Autodesk Fusion 360 part; units mm, degrees
(part 4 of 18)
  spline S17 degree 5 poles (4.4666, -33.3018) (4.4679, -33.2978) (4.4703, -33.2898) (4.474, -33.2778) (4.4789, -33.2619) (4.485, -33.242) (4.491, -33.2221) (4.497, -33.2023) (4.503, -33.1825) (4.5089, -33.1627) (4.5147, -33.1429) (4.5206, -33.1232) (4.5263, -33.1036) (4.5321, -33.0839) (4.5378, -33.0643) (4.5434, -33.0447) (4.549, -33.0252) (4.5546, -33.0057) (4.5601, -32.9862) (4.5656, -32.9667) (4.5711, -32.9473) (4.5765, -32.928) (4.5818, -32.9086) (4.5872, -32.8893) (4.5924, -32.87) (4.5977, -32.8508) (4.6029, -32.8316) (4.608, -32.8125) (4.6132, -32.7933) (4.6182, -32.7742) (4.6233, -32.7552) (4.6283, -32.7362) (4.6332, -32.7172) (4.6381, -32.6982) (4.643, -32.6793) (4.6478, -32.6605) (4.6526, -32.6416) (4.6574, -32.6228) (4.6621, -32.6041) (4.6667, -32.5854) (4.6714, -32.5667) (4.676, -32.5481) (4.6805, -32.5295) (4.685, -32.5109) (4.6895, -32.4924) (4.6939, -32.4739) (4.6983, -32.4555) (4.7026, -32.4371) (4.707, -32.4187) (4.7112, -32.4004) (4.7154, -32.3821) (4.7196, -32.3639) (4.7238, -32.3457) (4.7279, -32.3275) (4.732, -32.3094) (4.736, -32.2913) (4.74, -32.2733) (4.7439, -32.2553) (4.7478, -32.2374) (4.7517, -32.2195) (4.7555, -32.2016) (4.7593, -32.1838) (4.7631, -32.166) (4.7668, -32.1483) (4.7705, -32.1306) (4.7741, -32.113) (4.7777, -32.0954) (4.7813, -32.0779) (4.7848, -32.0604) (4.7883, -32.0429) (4.7917, -32.0255) (4.7951, -32.0081) (4.7985, -31.9908) (4.8018, -31.9736) (4.8051, -31.9563) (4.8083, -31.9392) (4.8115, -31.922) (4.8147, -31.905) (4.8179, -31.8879) (4.821, -31.871) (4.824, -31.854) (4.827, -31.8371) (4.83, -31.8203) (4.833, -31.8035) (4.8359, -31.7868) (4.8387, -31.7701) (4.8416, -31.7535) (4.8444, -31.7369) (4.8471, -31.7204) (4.8499, -31.7039) (4.8526, -31.6874) (4.8552, -31.6711) (4.8578, -31.6548) (4.8604, -31.6385) (4.8629, -31.6223) (4.8654, -31.6061) (4.8679, -31.59) (4.8703, -31.5739) (4.8727, -31.5579) (4.8751, -31.542) (4.8774, -31.5261) (4.8797, -31.5103) (4.882, -31.4945) (4.8842, -31.4787) (4.8864, -31.4631) (4.8885, -31.4475) (4.8906, -31.4319) (4.8927, -31.4164) (4.8947, -31.401) (4.8967, -31.3856) (4.8987, -31.3703) (4.9006, -31.355) (4.9026, -31.3398) (4.9044, -31.3247) (4.9063, -31.3096) (4.908, -31.2946) (4.9098, -31.2796) (4.9115, -31.2647) (4.9132, -31.2499) (4.9149, -31.2351) (4.9165, -31.2204) (4.9181, -31.2057) (4.9197, -31.1911) (4.9212, -31.1766) (4.9227, -31.1621) (4.9242, -31.1477) (4.9256, -31.1334) (4.927, -31.1191) (4.9284, -31.1049) (4.9297, -31.0908) (4.931, -31.0767) (4.9323, -31.0627) (4.9335, -31.0488) (4.9347, -31.0349) (4.9359, -31.0211) (4.9371, -31.0074) (4.9382, -30.9938) (4.9393, -30.9802) (4.9403, -30.9667) (4.9413, -30.9532) (4.9423, -30.9398) (4.9433, -30.9265) (4.9442, -30.9133) (4.9451, -30.9002) (4.946, -30.8871) (4.9468, -30.8741) (4.9476, -30.8611) (4.9484, -30.8483) (4.9492, -30.8355) (4.9499, -30.8228) (4.9506, -30.8102) (4.9513, -30.7976) (4.9519, -30.7851) (4.9525, -30.7727) (4.9531, -30.7604) (4.9537, -30.7482) (4.9542, -30.736) (4.9547, -30.724) (4.9552, -30.712) (4.9556, -30.7001) (4.9561, -30.6882) (4.9565, -30.6765) (4.9568, -30.6648) (4.9572, -30.6533) (4.9575, -30.6418) (4.9578, -30.6304) (4.9581, -30.6191) (4.9583, -30.6078) (4.9585, -30.5967) (4.9587, -30.5856) (4.9589, -30.5747) (4.9591, -30.5638) (4.9592, -30.553) (4.9593, -30.5424) (4.9594, -30.5318) (4.9594, -30.5213) (4.9595, -30.5109) (4.9595, -30.5006) (4.9595, -30.4904) (4.9595, -30.4802) (4.9594, -30.4702) (4.9594, -30.4603) (4.9593, -30.4505) (4.9592, -30.4408) (4.9591, -30.4312) (4.9589, -30.4217) (4.9588, -30.4122) (4.9586, -30.4029) (4.9584, -30.3938) (4.9582, -30.3847) (4.9579, -30.3757) (4.9577, -30.3668) (4.9574, -30.3581) (4.9572, -30.3494) (4.9569, -30.3409) (4.9566, -30.3324) (4.9562, -30.3241) (4.9559, -30.3159) (4.9556, -30.3079) (4.9552, -30.2999) (4.9548, -30.2921) (4.9545, -30.2844) (4.9541, -30.2768) (4.9537, -30.2693) (4.9532, -30.262) (4.9528, -30.2547) (4.9524, -30.2477) (4.9519, -30.2407) (4.9515, -30.2339) (4.951, -30.2272) (4.9506, -30.2206) (4.9501, -30.2142) (4.9496, -30.2079) (4.9492, -30.2018) (4.9487, -30.1958) (4.9482, -30.1899) (4.9477, -30.1842) (4.9472, -30.1787) (4.9468, -30.1733) (4.9463, -30.168) (4.9458, -30.1629) (4.9453, -30.158) (4.9448, -30.1532) (4.9444, -30.1486) (4.9439, -30.1441) (4.9434, -30.1398) (4.943, -30.1357) (4.9426, -30.1317) (4.9421, -30.128) (4.9417, -30.1244) (4.9413, -30.121) (4.9409, -30.1177) (4.9405, -30.1147) (4.9401, -30.1119) (4.9398, -30.1092) (4.9395, -30.1068) (4.9392, -30.1045) (4.9389, -30.1025) (4.9386, -30.1006) (4.9384, -30.099) (4.9382, -30.0976) (4.9381, -30.0967) (4.938, -30.0961) (4.9379, -30.0958) (4.9379, -30.0956) knots -1 -1 -1 -1 -1 -1 -0.99583333 -0.99166667 -0.9875 -0.98333333 -0.97916667 -0.975 -0.97083333 -0.96666667 -0.9625 -0.95833333 -0.95416667 -0.95 -0.94583333 -0.94166667 -0.9375 -0.93333333 -0.92916667 -0.925 -0.92083333 -0.91666667 -0.9125 -0.90833333 -0.90416667 -0.9 -0.89583333 -0.89166667 -0.8875 -0.88333333 -0.87916667 -0.875 -0.87083333 -0.86666667 -0.8625 -0.85833333 -0.85416667 -0.85 -0.84583333 -0.84166667 -0.8375 -0.83333333 -0.82916667 -0.825 -0.82083333 -0.81666667 -0.8125 -0.80833333 -0.80416667 -0.8 -0.79583333 -0.79166667 -0.7875 -0.78333333 -0.77916667 -0.775 -0.77083333 -0.76666667 -0.7625 -0.75833333 -0.75416667 -0.75 -0.74583333 -0.74166667 -0.7375 -0.73333333 -0.72916667 -0.725 -0.72083333 -0.71666667 -0.7125 -0.70833333 -0.70416667 -0.7 -0.69583333 -0.69166667 -0.6875 -0.68333333 -0.67916667 -0.675 -0.67083333 -0.66666667 -0.6625 -0.65833333 -0.65416667 -0.65 -0.64583333 -0.64166667 -0.6375 -0.63333333 -0.62916667 -0.625 -0.62083333 -0.61666667 -0.6125 -0.60833333 -0.60416667 -0.6 -0.59583333 -0.59166667 -0.5875 -0.58333333 -0.57916667 -0.575 -0.57083333 -0.56666667 -0.5625 -0.55833333 -0.55416667 -0.55 -0.54583333 -0.54166667 -0.5375 -0.53333333 -0.52916667 -0.525 -0.52083333 -0.51666667 -0.5125 -0.50833333 -0.50416667 -0.5 -0.49583333 -0.49166667 -0.4875 -0.48333333 -0.47916667 -0.475 -0.47083333 -0.46666667 -0.4625 -0.45833333 -0.45416667 -0.45 -0.44583333 -0.44166667 -0.4375 -0.43333333 -0.42916667 -0.425 -0.42083333 -0.41666667 -0.4125 -0.40833333 -0.40416667 -0.4 -0.39583333 -0.39166667 -0.3875 -0.38333333 -0.37916667 -0.375 -0.37083333 -0.36666667 -0.3625 -0.35833333 -0.35416667 -0.35 -0.34583333 -0.34166667 -0.3375 -0.33333333 -0.32916667 -0.325 -0.32083333 -0.31666667 -0.3125 -0.30833333 -0.30416667 -0.3 -0.29583333 -0.29166667 -0.2875 -0.28333333 -0.27916667 -0.275 -0.27083333 -0.26666667 -0.2625 -0.25833333 -0.25416667 -0.25 -0.24583333 -0.24166667 -0.2375 -0.23333333 -0.22916667 -0.225 -0.22083333 -0.21666667 -0.2125 -0.20833333 -0.20416667 -0.2 -0.19583333 -0.19166667 -0.1875 -0.18333333 -0.17916667 -0.175 -0.17083333 -0.16666667 -0.1625 -0.15833333 -0.15416667 -0.15 -0.14583333 -0.14166667 -0.1375 -0.13333333 -0.12916667 -0.125 -0.12083333 -0.11666667 -0.1125 -0.10833333 -0.10416667 -0.1 -0.09583333 -0.09166667 -0.0875 -0.08333333 -0.07916667 -0.075 -0.07083333 -0.06666667 -0.0625 -0.05833333 -0.05416667 -0.05 -0.04583333 -0.04166667 -0.0375 -0.03333333 -0.02916667 -0.025 -0.02083333 -0.01666667 -0.0125 -0.00833333 -0.00416667 0 0 0 0 0 0
  line L34 (4.9379, -30.0956) -> (4.9377, -30.0943)
  line L35 (4.9377, -30.0943) -> (4.6751, -28.494)
  arc A18 (4.6751, -28.494) -> (7.3186, -27.9321) centre (0, 0) ccw
  line L36 (7.3186, -27.9321) -> (7.7297, -29.5008)
  line L37 (7.7297, -29.5008) -> (7.73, -29.5021)
  spline S18 degree 5 poles (7.73, -29.5021) (7.7301, -29.5023) (7.7301, -29.5026) (7.7303, -29.5032) (7.7306, -29.5041) (7.7309, -29.5055) (7.7314, -29.507) (7.7319, -29.5088) (7.7325, -29.5108) (7.7331, -29.513) (7.7338, -29.5153) (7.7345, -29.5179) (7.7354, -29.5206) (7.7363, -29.5236) (7.7372, -29.5267) (7.7382, -29.53) (7.7393, -29.5334) (7.7404, -29.537) (7.7416, -29.5408) (7.7429, -29.5448) (7.7442, -29.5489) (7.7456, -29.5531) (7.7471, -29.5576) (7.7486, -29.5621) (7.7502, -29.5668) (7.7518, -29.5717) (7.7535, -29.5767) (7.7552, -29.5818) (7.7571, -29.5871) (7.7589, -29.5925) (7.7609, -29.598) (7.7629, -29.6037) (7.765, -29.6095) (7.7671, -29.6155) (7.7693, -29.6215) (7.7715, -29.6277) (7.7738, -29.634) (7.7762, -29.6404) (7.7786, -29.6469) (7.7811, -29.6536) (7.7836, -29.6603) (7.7862, -29.6672) (7.7889, -29.6742) (7.7916, -29.6813) (7.7944, -29.6885) (7.7973, -29.6958) (7.8002, -29.7032) (7.8032, -29.7107) (7.8062, -29.7184) (7.8093, -29.7261) (7.8124, -29.7339) (7.8156, -29.7418) (7.8189, -29.7498) (7.8222, -29.7579) (7.8256, -29.7661) (7.829, -29.7744) (7.8325, -29.7828) (7.8361, -29.7913) (7.8397, -29.7999) (7.8434, -29.8085) (7.8471, -29.8173) (7.8509, -29.8261) (7.8548, -29.835) (7.8587, -29.844) (7.8627, -29.8531) (7.8667, -29.8623) (7.8708, -29.8715) (7.875, -29.8809) (7.8792, -29.8903) (7.8834, -29.8998) (7.8878, -29.9093) (7.8922, -29.919) (7.8966, -29.9287) (7.9011, -29.9385) (7.9057, -29.9483) (7.9103, -29.9583) (7.9149, -29.9683) (7.9197, -29.9784) (7.9245, -29.9885) (7.9293, -29.9988) (7.9342, -30.0091) (7.9392, -30.0194) (7.9442, -30.0298) (7.9493, -30.0403) (7.9544, -30.0509) (7.9596, -30.0615) (7.9649, -30.0722) (7.9702, -30.083) (7.9756, -30.0938) (7.981, -30.1047) (7.9865, -30.1157) (7.992, -30.1267) (7.9976, -30.1378) (8.0033, -30.1489) (8.009, -30.1601) (8.0148, -30.1713) (8.0206, -30.1826) (8.0265, -30.194) (8.0325, -30.2054) (8.0385, -30.2169) (8.0445, -30.2285) (8.0506, -30.2401) (8.0568, -30.2517) (8.063, -30.2634) (8.0693, -30.2752) (8.0757, -30.287) (8.0821, -30.2989) (8.0885, -30.3108) (8.0951, -30.3228) (8.1016, -30.3348) (8.1083, -30.3468) (8.1149, -30.359) (8.1217, -30.3711) (8.1285, -30.3834) (8.1353, -30.3956) (8.1422, -30.408) (8.1492, -30.4203) (8.1562, -30.4327) (8.1633, -30.4452) (8.1705, -30.4577) (8.1776, -30.4703) (8.1849, -30.4829) (8.1922, -30.4955) (8.1996, -30.5082) (8.207, -30.521) (8.2145, -30.5337) (8.222, -30.5466) (8.2296, -30.5594) (8.2372, -30.5723) (8.2449, -30.5853) (8.2527, -30.5983) (8.2605, -30.6113) (8.2683, -30.6244) (8.2763, -30.6375) (8.2842, -30.6507) (8.2923, -30.6639) (8.3004, -30.6771) (8.3085, -30.6904) (8.3167, -30.7037) (8.325, -30.717) (8.3333, -30.7304) (8.3416, -30.7438) (8.3501, -30.7573) (8.3585, -30.7708) (8.3671, -30.7843) (8.3757, -30.7979) (8.3843, -30.8115) (8.393, -30.8252) (8.4017, -30.8388) (8.4106, -30.8526) (8.4194, -30.8663) (8.4283, -30.8801) (8.4373, -30.8939) (8.4463, -30.9078) (8.4554, -30.9216) (8.4646, -30.9356) (8.4737, -30.9495) (8.483, -30.9635) (8.4923, -30.9775) (8.5016, -30.9915) (8.5111, -31.0056) (8.5205, -31.0197) (8.53, -31.0338) (8.5396, -31.048) (8.5492, -31.0622) (8.5589, -31.0764) (8.5687, -31.0907) (8.5785, -31.105) (8.5883, -31.1193) (8.5982, -31.1336) (8.6082, -31.148) (8.6182, -31.1624) (8.6282, -31.1768) (8.6383, -31.1912) (8.6485, -31.2057) (8.6587, -31.2202) (8.669, -31.2348) (8.6794, -31.2493) (8.6897, -31.2639) (8.7002, -31.2785) (8.7107, -31.2931) (8.7212, -31.3078) (8.7318, -31.3225) (8.7425, -31.3372) (8.7532, -31.3519) (8.7639, -31.3667) (8.7748, -31.3814) (8.7856, -31.3962) (8.7966, -31.4111) (8.8075, -31.4259) (8.8186, -31.4408) (8.8296, -31.4557) (8.8408, -31.4706) (8.852, -31.4855) (8.8632, -31.5005) (8.8745, -31.5154) (8.8859, -31.5304) (8.8973, -31.5455) (8.9087, -31.5605) (8.9202, -31.5756) (8.9318, -31.5907) (8.9434, -31.6058) (8.9551, -31.6209) (8.9668, -31.636) (8.9786, -31.6512) (8.9904, -31.6664) (9.0023, -31.6816) (9.0142, -31.6968) (9.0262, -31.712) (9.0382, -31.7273) (9.0503, -31.7425) (9.0624, -31.7578) (9.0746, -31.7731) (9.0869, -31.7885) (9.0992, -31.8038) (9.1115, -31.8192) (9.1239, -31.8345) (9.1364, -31.8499) (9.1489, -31.8653) (9.1614, -31.8808) (9.174, -31.8962) (9.1867, -31.9117) (9.1994, -31.9271) (9.2122, -31.9426) (9.225, -31.9581) (9.2379, -31.9736) (9.2508, -31.9892) (9.2638, -32.0047) (9.2768, -32.0203) (9.2899, -32.0358) (9.303, -32.0514) (9.3162, -32.067) (9.3294, -32.0826) (9.3427, -32.0982) (9.356, -32.1139) (9.3694, -32.1295) (9.3829, -32.1452) (9.3964, -32.1609) (9.4099, -32.1766) (9.4235, -32.1923) (9.4371, -32.208) (9.4481, -32.2206) (9.4563, -32.23) (9.4618, -32.2363) (9.4646, -32.2394) knots 0 0 0 0 0 0 0.00416667 0.00833333 0.0125 0.01666667 0.02083333 0.025 0.02916667 0.03333333 0.0375 0.04166667 0.04583333 0.05 0.05416667 0.05833333 0.0625 0.06666667 0.07083333 0.075 0.07916667 0.08333333 0.0875 0.09166667 0.09583333 0.1 0.10416667 0.10833333 0.1125 0.11666667 0.12083333 0.125 0.12916667 0.13333333 0.1375 0.14166667 0.14583333 0.15 0.15416667 0.15833333 0.1625 0.16666667 0.17083333 0.175 0.17916667 0.18333333 0.1875 0.19166667 0.19583333 0.2 0.20416667 0.20833333 0.2125 0.21666667 0.22083333 0.225 0.22916667 0.23333333 0.2375 0.24166667 0.24583333 0.25 0.25416667 0.25833333 0.2625 0.26666667 0.27083333 0.275 0.27916667 0.28333333 0.2875 0.29166667 0.29583333 0.3 0.30416667 0.30833333 0.3125 0.31666667 0.32083333 0.325 0.32916667 0.33333333 0.3375 0.34166667 0.34583333 0.35 0.35416667 0.35833333 0.3625 0.36666667 0.37083333 0.375 0.37916667 0.38333333 0.3875 0.39166667 0.39583333 0.4 0.40416667 0.40833333 0.4125 0.41666667 0.42083333 0.425 0.42916667 0.43333333 0.4375 0.44166667 0.44583333 0.45 0.45416667 0.45833333 0.4625 0.46666667 0.47083333 0.475 0.47916667 0.48333333 0.4875 0.49166667 0.49583333 0.5 0.50416667 0.50833333 0.5125 0.51666667 0.52083333 0.525 0.52916667 0.53333333 0.5375 0.54166667 0.54583333 0.55 0.55416667 0.55833333 0.5625 0.56666667 0.57083333 0.575 0.57916667 0.58333333 0.5875 0.59166667 0.59583333 0.6 0.60416667 0.60833333 0.6125 0.61666667 0.62083333 0.625 0.62916667 0.63333333 0.6375 0.64166667 0.64583333 0.65 0.65416667 0.65833333 0.6625 0.66666667 0.67083333 0.675 0.67916667 0.68333333 0.6875 0.69166667 0.69583333 0.7 0.70416667 0.70833333 0.7125 0.71666667 0.72083333 0.725 0.72916667 0.73333333 0.7375 0.74166667 0.74583333 0.75 0.75416667 0.75833333 0.7625 0.76666667 0.77083333 0.775 0.77916667 0.78333333 0.7875 0.79166667 0.79583333 0.8 0.80416667 0.80833333 0.8125 0.81666667 0.82083333 0.825 0.82916667 0.83333333 0.8375 0.84166667 0.84583333 0.85 0.85416667 0.85833333 0.8625 0.86666667 0.87083333 0.875 0.87916667 0.88333333 0.8875 0.89166667 0.89583333 0.9 0.90416667 0.90833333 0.9125 0.91666667 0.92083333 0.925 0.92916667 0.93333333 0.9375 0.94166667 0.94583333 0.95 0.95416667 0.95833333 0.9625 0.96666667 0.97083333 0.975 0.97916667 0.98333333 0.9875 0.99166667 0.99583333 1 1 1 1 1 1
  arc A19 (9.4646, -32.2394) -> (11.2929, -31.6454) centre (0, 0) ccw
  spline S19 degree 5 poles (11.2929, -31.6454) (11.2932, -31.6412) (11.294, -31.6329) (11.2951, -31.6204) (11.2966, -31.6038) (11.2984, -31.5831) (11.3001, -31.5624) (11.3019, -31.5417) (11.3036, -31.5211) (11.3052, -31.5006) (11.3069, -31.48) (11.3085, -31.4595) (11.31, -31.4391) (11.3116, -31.4187) (11.3131, -31.3983) (11.3145, -31.378) (11.3159, -31.3577) (11.3173, -31.3375) (11.3187, -31.3173) (11.32, -31.2971) (11.3213, -31.277) (11.3226, -31.2569) (11.3238, -31.2369) (11.325, -31.2169) (11.3262, -31.1969) (11.3273, -31.177) (11.3284, -31.1572) (11.3294, -31.1374) (11.3305, -31.1176) (11.3315, -31.0979) (11.3324, -31.0782) (11.3334, -31.0585) (11.3343, -31.0389) (11.3351, -31.0194) (11.336, -30.9999) (11.3368, -30.9804) (11.3375, -30.961) (11.3383, -30.9416) (11.339, -30.9223) (11.3397, -30.903) (11.3403, -30.8838) (11.3409, -30.8646) (11.3415, -30.8455) (11.342, -30.8264) (11.3426, -30.8073) (11.343, -30.7884) (11.3435, -30.7694) (11.3439, -30.7505) (11.3443, -30.7316) (11.3447, -30.7128) (11.345, -30.6941) (11.3453, -30.6754) (11.3456, -30.6567) (11.3458, -30.6381) (11.3461, -30.6195) (11.3462, -30.601) (11.3464, -30.5826) (11.3465, -30.5642) (11.3466, -30.5458) (11.3467, -30.5275) (11.3467, -30.5092) (11.3467, -30.491) (11.3467, -30.4728) (11.3466, -30.4547) (11.3466, -30.4367) (11.3464, -30.4187) (11.3463, -30.4007) (11.3461, -30.3828) (11.3459, -30.365) (11.3457, -30.3472) (11.3455, -30.3294) (11.3452, -30.3117) (11.3449, -30.2941) (11.3445, -30.2765) (11.3442, -30.259) (11.3438, -30.2415) (11.3434, -30.2241) (11.3429, -30.2067) (11.3424, -30.1894) (11.3419, -30.1722) (11.3414, -30.155) (11.3409, -30.1378) (11.3403, -30.1207) (11.3397, -30.1037) (11.339, -30.0867) (11.3384, -30.0698) (11.3377, -30.053) (11.337, -30.0362) (11.3363, -30.0194) (11.3355, -30.0027) (11.3347, -29.9861) (11.3339, -29.9695) (11.3331, -29.953) (11.3322, -29.9366) (11.3313, -29.9202) (11.3304, -29.9038) (11.3295, -29.8876) (11.3285, -29.8714) (11.3275, -29.8552) (11.3265, -29.8391) (11.3255, -29.8231) (11.3244, -29.8071) (11.3234, -29.7912) (11.3222, -29.7754) (11.3211, -29.7596) (11.32, -29.7439) (11.3188, -29.7282) (11.3176, -29.7126) (11.3164, -29.6971) (11.3152, -29.6817) (11.3139, -29.6663) (11.3126, -29.6509) (11.3113, -29.6357) (11.31, -29.6205) (11.3087, -29.6053) (11.3073, -29.5903) (11.3059, -29.5753) (11.3045, -29.5603) (11.3031, -29.5454) (11.3016, -29.5306) (11.3002, -29.5159) (11.2987, -29.5013) (11.2972, -29.4867) (11.2957, -29.4721) (11.2941, -29.4577) (11.2926, -29.4433) (11.291, -29.429) (11.2894, -29.4147) (11.2878, -29.4006) (11.2861, -29.3865) (11.2845, -29.3724) (11.2828, -29.3585) (11.2811, -29.3446) (11.2794, -29.3308) (11.2777, -29.317) (11.276, -29.3034) (11.2742, -29.2898) (11.2725, -29.2763) (11.2707, -29.2628) (11.2689, -29.2495) (11.2671, -29.2362) (11.2653, -29.223) (11.2634, -29.2098) (11.2616, -29.1968) (11.2597, -29.1838) (11.2578, -29.1709) (11.2559, -29.1581) (11.254, -29.1453) (11.2521, -29.1327) (11.2502, -29.1201) (11.2482, -29.1076) (11.2463, -29.0952) (11.2443, -29.0829) (11.2423, -29.0706) (11.2403, -29.0584) (11.2383, -29.0464) (11.2363, -29.0344) (11.2343, -29.0224) (11.2323, -29.0106) (11.2302, -28.9989) (11.2282, -28.9872) (11.2261, -28.9756) (11.2241, -28.9642) (11.222, -28.9528) (11.2199, -28.9415) (11.2179, -28.9302) (11.2158, -28.9191) (11.2137, -28.9081) (11.2116, -28.8971) (11.2095, -28.8863) (11.2074, -28.8755) (11.2053, -28.8649) (11.2032, -28.8543) (11.201, -28.8438) (11.1989, -28.8335) (11.1968, -28.8232) (11.1947, -28.813) (11.1926, -28.8029) (11.1904, -28.7929) (11.1883, -28.783) (11.1862, -28.7733) (11.1841, -28.7636) (11.1819, -28.754) (11.1798, -28.7445) (11.1777, -28.7351) (11.1756, -28.7259) (11.1735, -28.7167) (11.1714, -28.7076) (11.1693, -28.6987) (11.1672, -28.6898) (11.1651, -28.6811) (11.163, -28.6725) (11.1609, -28.6639) (11.1588, -28.6555) (11.1568, -28.6473) (11.1547, -28.6391) (11.1527, -28.631) (11.1507, -28.6231) (11.1486, -28.6153) (11.1466, -28.6075) (11.1446, -28.6) (11.1427, -28.5925) (11.1407, -28.5851) (11.1387, -28.5779) (11.1368, -28.5708) (11.1349, -28.5639) (11.133, -28.557) (11.1311, -28.5503) (11.1293, -28.5437) (11.1274, -28.5373) (11.1256, -28.531) (11.1238, -28.5248) (11.1221, -28.5187) (11.1203, -28.5128) (11.1186, -28.5071) (11.1169, -28.5014) (11.1153, -28.496) (11.1136, -28.4906) (11.112, -28.4854) (11.1105, -28.4804) (11.1089, -28.4755) (11.1074, -28.4708) (11.106, -28.4662) (11.1046, -28.4618) (11.1032, -28.4575) (11.1018, -28.4534) (11.1005, -28.4495) (11.0993, -28.4457) (11.0981, -28.4421) (11.0969, -28.4387) (11.0958, -28.4354) (11.0948, -28.4323) (11.0937, -28.4294) (11.0928, -28.4267) (11.0919, -28.4242) (11.0911, -28.4219) (11.0903, -28.4197) (11.0896, -28.4178) (11.089, -28.4161) (11.0884, -28.4145) (11.0879, -28.4132) (11.0876, -28.4124) (11.0874, -28.4118) (11.0873, -28.4115) (11.0872, -28.4113) knots -1 -1 -1 -1 -1 -1 -0.99583333 -0.99166667 -0.9875 -0.98333333 -0.97916667 -0.975 -0.97083333 -0.96666667 -0.9625 -0.95833333 -0.95416667 -0.95 -0.94583333 -0.94166667 -0.9375 -0.93333333 -0.92916667 -0.925 -0.92083333 -0.91666667 -0.9125 -0.90833333 -0.90416667 -0.9 -0.89583333 -0.89166667 -0.8875 -0.88333333 -0.87916667 -0.875 -0.87083333 -0.86666667 -0.8625 -0.85833333 -0.85416667 -0.85 -0.84583333 -0.84166667 -0.8375 -0.83333333 -0.82916667 -0.825 -0.82083333 -0.81666667 -0.8125 -0.80833333 -0.80416667 -0.8 -0.79583333 -0.79166667 -0.7875 -0.78333333 -0.77916667 -0.775 -0.77083333 -0.76666667 -0.7625 -0.75833333 -0.75416667 -0.75 -0.74583333 -0.74166667 -0.7375 -0.73333333 -0.72916667 -0.725 -0.72083333 -0.71666667 -0.7125 -0.70833333 -0.70416667 -0.7 -0.69583333 -0.69166667 -0.6875 -0.68333333 -0.67916667 -0.675 -0.67083333 -0.66666667 -0.6625 -0.65833333 -0.65416667 -0.65 -0.64583333 -0.64166667 -0.6375 -0.63333333 -0.62916667 -0.625 -0.62083333 -0.61666667 -0.6125 -0.60833333 -0.60416667 -0.6 -0.59583333 -0.59166667 -0.5875 -0.58333333 -0.57916667 -0.575 -0.57083333 -0.56666667 -0.5625 -0.55833333 -0.55416667 -0.55 -0.54583333 -0.54166667 -0.5375 -0.53333333 -0.52916667 -0.525 -0.52083333 -0.51666667 -0.5125 -0.50833333 -0.50416667 -0.5 -0.49583333 -0.49166667 -0.4875 -0.48333333 -0.47916667 -0.475 -0.47083333 -0.46666667 -0.4625 -0.45833333 -0.45416667 -0.45 -0.44583333 -0.44166667 -0.4375 -0.43333333 -0.42916667 -0.425 -0.42083333 -0.41666667 -0.4125 -0.40833333 -0.40416667 -0.4 -0.39583333 -0.39166667 -0.3875 -0.38333333 -0.37916667 -0.375 -0.37083333 -0.36666667 -0.3625 -0.35833333 -0.35416667 -0.35 -0.34583333 -0.34166667 -0.3375 -0.33333333 -0.32916667 -0.325 -0.32083333 -0.31666667 -0.3125 -0.30833333 -0.30416667 -0.3 -0.29583333 -0.29166667 -0.2875 -0.28333333 -0.27916667 -0.275 -0.27083333 -0.26666667 -0.2625 -0.25833333 -0.25416667 -0.25 -0.24583333 -0.24166667 -0.2375 -0.23333333 -0.22916667 -0.225 -0.22083333 -0.21666667 -0.2125 -0.20833333 -0.20416667 -0.2 -0.19583333 -0.19166667 -0.1875 -0.18333333 -0.17916667 -0.175 -0.17083333 -0.16666667 -0.1625 -0.15833333 -0.15416667 -0.15 -0.14583333 -0.14166667 -0.1375 -0.13333333 -0.12916667 -0.125 -0.12083333 -0.11666667 -0.1125 -0.10833333 -0.10416667 -0.1 -0.09583333 -0.09166667 -0.0875 -0.08333333 -0.07916667 -0.075 -0.07083333 -0.06666667 -0.0625 -0.05833333 -0.05416667 -0.05 -0.04583333 -0.04166667 -0.0375 -0.03333333 -0.02916667 -0.025 -0.02083333 -0.01666667 -0.0125 -0.00833333 -0.00416667 0 0 0 0 0 0
  line L38 (11.0872, -28.4113) -> (11.0867, -28.41)
  line L39 (11.0867, -28.41) -> (10.4972, -26.8993)
  arc A20 (10.4972, -26.8993) -> (12.9661, -25.8001) centre (0, 0) ccw
  line L40 (12.9661, -25.8001) -> (13.6943, -27.2491)
  line L41 (13.6943, -27.2491) -> (13.6949, -27.2503)
  spline S20 degree 5 poles (13.6949, -27.2503) (13.695, -27.2504) (13.6952, -27.2507) (13.6954, -27.2513) (13.6959, -27.2521) (13.6965, -27.2533) (13.6973, -27.2548) (13.6981, -27.2564) (13.6991, -27.2582) (13.7002, -27.2602) (13.7014, -27.2624) (13.7026, -27.2647) (13.704, -27.2673) (13.7055, -27.2699) (13.7071, -27.2728) (13.7087, -27.2758) (13.7105, -27.2789) (13.7124, -27.2823) (13.7144, -27.2857) (13.7164, -27.2893) (13.7186, -27.293) (13.7208, -27.2969) (13.7231, -27.3009) (13.7256, -27.3051) (13.7281, -27.3094) (13.7307, -27.3138) (13.7334, -27.3183) (13.7362, -27.323) (13.7391, -27.3278) (13.742, -27.3327) (13.7451, -27.3377) (13.7482, -27.3428) (13.7514, -27.3481) (13.7547, -27.3534) (13.7581, -27.3589) (13.7616, -27.3645) (13.7652, -27.3701) (13.7688, -27.3759) (13.7726, -27.3818) (13.7764, -27.3878) (13.7803, -27.3939) (13.7843, -27.4001) (13.7883, -27.4063) (13.7925, -27.4127) (13.7967, -27.4192) (13.801, -27.4257) (13.8054, -27.4324) (13.8098, -27.4391) (13.8144, -27.446) (13.819, -27.4529) (13.8237, -27.4599) (13.8285, -27.4669) (13.8334, -27.4741) (13.8383, -27.4813) (13.8433, -27.4887) (13.8484, -27.4961) (13.8536, -27.5035) (13.8588, -27.5111) (13.8641, -27.5187) (13.8695, -27.5264) (13.875, -27.5342) (13.8806, -27.542) (13.8862, -27.55) (13.8919, -27.558) (13.8977, -27.566) (13.9035, -27.5741) (13.9095, -27.5823) (13.9155, -27.5906) (13.9215, -27.5989) (13.9277, -27.6073) (13.9339, -27.6158) (13.9402, -27.6243) (13.9466, -27.6329) (13.953, -27.6415) (13.9595, -27.6502) (13.9661, -27.659) (13.9727, -27.6678) (13.9795, -27.6767) (13.9863, -27.6856) (13.9931, -27.6946) (14.0001, -27.7037) (14.0071, -27.7128) (14.0142, -27.7219) (14.0213, -27.7311) (14.0286, -27.7404) (14.0359, -27.7497) (14.0432, -27.7591) (14.0507, -27.7685) (14.0582, -27.778) (14.0657, -27.7875) (14.0734, -27.7971) (14.0811, -27.8067) (14.0889, -27.8164) (14.0967, -27.8261) (14.1046, -27.8358) (14.1126, -27.8456) (14.1207, -27.8555) (14.1288, -27.8654) (14.137, -27.8753) (14.1453, -27.8853) (14.1536, -27.8954) (14.162, -27.9054) (14.1704, -27.9155) (14.179, -27.9257) (14.1876, -27.9359) (14.1962, -27.9461) (14.205, -27.9564) (14.2137, -27.9667) (14.2226, -27.9771) (14.2315, -27.9875) (14.2405, -27.9979) (14.2496, -28.0084) (14.2587, -28.0189) (14.2679, -28.0294) (14.2772, -28.04) (14.2865, -28.0506) (14.2959, -28.0613) (14.3053, -28.0719) (14.3148, -28.0827) (14.3244, -28.0934) (14.3341, -28.1042) (14.3438, -28.115) (14.3536, -28.1259) (14.3634, -28.1368) (14.3733, -28.1477) (14.3833, -28.1586) (14.3933, -28.1696) (14.4034, -28.1806) (14.4136, -28.1916) (14.4238, -28.2027) (14.4341, -28.2138) (14.4444, -28.2249) (14.4548, -28.2361) (14.4653, -28.2473) (14.4758, -28.2585) (14.4864, -28.2697) (14.4971, -28.281) (14.5078, -28.2923) (14.5186, -28.3036) (14.5295, -28.3149) (14.5404, -28.3263) (14.5514, -28.3377) (14.5624, -28.3491) (14.5735, -28.3606) (14.5847, -28.372) (14.5959, -28.3835) (14.6072, -28.395) (14.6185, -28.4066) (14.6299, -28.4181) (14.6414, -28.4297) (14.6529, -28.4413) (14.6645, -28.4529) (14.6761, -28.4646) (14.6878, -28.4763) (14.6996, -28.4879) (14.7114, -28.4997) (14.7233, -28.5114) (14.7353, -28.5231) (14.7473, -28.5349) (14.7594, -28.5467) (14.7715, -28.5585) (14.7837, -28.5703) (14.7959, -28.5822) (14.8083, -28.594) (14.8206, -28.6059) (14.833, -28.6178) (14.8455, -28.6297) (14.8581, -28.6417) (14.8707, -28.6536) (14.8834, -28.6656) (14.8961, -28.6776) (14.9089, -28.6896) (14.9217, -28.7016) (14.9346, -28.7136) (14.9476, -28.7257) (14.9606, -28.7377) (14.9737, -28.7498) (14.9868, -28.7619) (15, -28.774) (15.0132, -28.7861) (15.0265, -28.7982) (15.0399, -28.8104) (15.0533, -28.8225) (15.0668, -28.8347) (15.0803, -28.8469) (15.0939, -28.8591) (15.1076, -28.8713) (15.1213, -28.8835) (15.1351, -28.8957) (15.1489, -28.908) (15.1628, -28.9202) (15.1767, -28.9325) (15.1907, -28.9448) (15.2047, -28.9571) (15.2188, -28.9693) (15.233, -28.9816) (15.2472, -28.994) (15.2615, -29.0063) (15.2758, -29.0186) (15.2902, -29.031) (15.3047, -29.0433) (15.3192, -29.0557) (15.3337, -29.068) (15.3483, -29.0804) (15.363, -29.0928) (15.3777, -29.1052) (15.3925, -29.1176) (15.4073, -29.13) (15.4222, -29.1424) (15.4372, -29.1548) (15.4522, -29.1672) (15.4672, -29.1797) (15.4823, -29.1921) (15.4975, -29.2045) (15.5127, -29.217) (15.528, -29.2294) (15.5433, -29.2419) (15.5587, -29.2544) (15.5741, -29.2668) (15.5896, -29.2793) (15.6052, -29.2918) (15.6208, -29.3043) (15.6364, -29.3168) (15.6521, -29.3293) (15.6679, -29.3418) (15.6837, -29.3543) (15.6996, -29.3668) (15.7155, -29.3793) (15.7315, -29.3918) (15.7475, -29.4043) (15.7636, -29.4168) (15.7797, -29.4293) (15.7959, -29.4418) (15.8121, -29.4544) (15.8284, -29.4669) (15.8448, -29.4794) (15.8612, -29.4919) (15.8776, -29.5045) (15.8941, -29.517) (15.9107, -29.5295) (15.9273, -29.5421) (15.9406, -29.5521) (15.9507, -29.5596) (15.9574, -29.5646) (15.9607, -29.5671) knots 0 0 0 0 0 0 0.00416667 0.00833333 0.0125 0.01666667 0.02083333 0.025 0.02916667 0.03333333 0.0375 0.04166667 0.04583333 0.05 0.05416667 0.05833333 0.0625 0.06666667 0.07083333 0.075 0.07916667 0.08333333 0.0875 0.09166667 0.09583333 0.1 0.10416667 0.10833333 0.1125 0.11666667 0.12083333 0.125 0.12916667 0.13333333 0.1375 0.14166667 0.14583333 0.15 0.15416667 0.15833333 0.1625 0.16666667 0.17083333 0.175 0.17916667 0.18333333 0.1875 0.19166667 0.19583333 0.2 0.20416667 0.20833333 0.2125 0.21666667 0.22083333 0.225 0.22916667 0.23333333 0.2375 0.24166667 0.24583333 0.25 0.25416667 0.25833333 0.2625 0.26666667 0.27083333 0.275 0.27916667 0.28333333 0.2875 0.29166667 0.29583333 0.3 0.30416667 0.30833333 0.3125 0.31666667 0.32083333 0.325 0.32916667 0.33333333 0.3375 0.34166667 0.34583333 0.35 0.35416667 0.35833333 0.3625 0.36666667 0.37083333 0.375 0.37916667 0.38333333 0.3875 0.39166667 0.39583333 0.4 0.40416667 0.40833333 0.4125 0.41666667 0.42083333 0.425 0.42916667 0.43333333 0.4375 0.44166667 0.44583333 0.45 0.45416667 0.45833333 0.4625 0.46666667 0.47083333 0.475 0.47916667 0.48333333 0.4875 0.49166667 0.49583333 0.5 0.50416667 0.50833333 0.5125 0.51666667 0.52083333 0.525 0.52916667 0.53333333 0.5375 0.54166667 0.54583333 0.55 0.55416667 0.55833333 0.5625 0.56666667 0.57083333 0.575 0.57916667 0.58333333 0.5875 0.59166667 0.59583333 0.6 0.60416667 0.60833333 0.6125 0.61666667 0.62083333 0.625 0.62916667 0.63333333 0.6375 0.64166667 0.64583333 0.65 0.65416667 0.65833333 0.6625 0.66666667 0.67083333 0.675 0.67916667 0.68333333 0.6875 0.69166667 0.69583333 0.7 0.70416667 0.70833333 0.7125 0.71666667 0.72083333 0.725 0.72916667 0.73333333 0.7375 0.74166667 0.74583333 0.75 0.75416667 0.75833333 0.7625 0.76666667 0.77083333 0.775 0.77916667 0.78333333 0.7875 0.79166667 0.79583333 0.8 0.80416667 0.80833333 0.8125 0.81666667 0.82083333 0.825 0.82916667 0.83333333 0.8375 0.84166667 0.84583333 0.85 0.85416667 0.85833333 0.8625 0.86666667 0.87083333 0.875 0.87916667 0.88333333 0.8875 0.89166667 0.89583333 0.9 0.90416667 0.90833333 0.9125 0.91666667 0.92083333 0.925 0.92916667 0.93333333 0.9375 0.94166667 0.94583333 0.95 0.95416667 0.95833333 0.9625 0.96666667 0.97083333 0.975 0.97916667 0.98333333 0.9875 0.99166667 0.99583333 1 1 1 1 1 1
  arc A21 (15.9607, -29.5671) -> (17.6255, -28.606) centre (0, 0) ccw
  spline S21 degree 5 poles (17.6255, -28.606) (17.625, -28.6018) (17.624, -28.5935) (17.6225, -28.5811) (17.6205, -28.5645) (17.618, -28.5438) (17.6154, -28.5232) (17.6128, -28.5027) (17.6102, -28.4822) (17.6075, -28.4617) (17.6049, -28.4413) (17.6022, -28.4209) (17.5994, -28.4006) (17.5967, -28.3803) (17.5939, -28.3601) (17.5911, -28.3399) (17.5883, -28.3197) (17.5854, -28.2996) (17.5826, -28.2796) (17.5797, -28.2596) (17.5768, -28.2397) (17.5738, -28.2198) (17.5709, -28.1999) (17.5679, -28.1801) (17.5649, -28.1604) (17.5618, -28.1407) (17.5588, -28.121) (17.5557, -28.1014) (17.5526, -28.0819) (17.5494, -28.0624) (17.5463, -28.0429) (17.5431, -28.0235) (17.5399, -28.0041) (17.5367, -27.9848) (17.5335, -27.9656) (17.5302, -27.9464) (17.5269, -27.9272) (17.5236, -27.9081) (17.5203, -27.8891) (17.517, -27.8701) (17.5136, -27.8511) (17.5102, -27.8322) (17.5068, -27.8134) (17.5034, -27.7946) (17.4999, -27.7759) (17.4964, -27.7572) (17.4929, -27.7386) (17.4894, -27.72) (17.4859, -27.7015) (17.4823, -27.683) (17.4788, -27.6646) (17.4752, -27.6462) (17.4716, -27.6279) (17.4679, -27.6097) (17.4643, -27.5915) (17.4606, -27.5733) (17.4569, -27.5552) (17.4532, -27.5372) (17.4495, -27.5192) (17.4457, -27.5013) (17.442, -27.4834) (17.4382, -27.4656) (17.4344, -27.4478) (17.4306, -27.4301) (17.4267, -27.4125) (17.4229, -27.3949) (17.419, -27.3774) (17.4151, -27.3599) (17.4112, -27.3425) (17.4073, -27.3251) (17.4034, -27.3078) (17.3994, -27.2906) (17.3955, -27.2734) (17.3915, -27.2562) (17.3875, -27.2392) (17.3835, -27.2222) (17.3794, -27.2052) (17.3754, -27.1883) (17.3713, -27.1715) (17.3672, -27.1547) (17.3632, -27.138) (17.359, -27.1213) (17.3549, -27.1048) (17.3508, -27.0882) (17.3466, -27.0717) (17.3425, -27.0553) (17.3383, -27.039) (17.3341, -27.0227) (17.3299, -27.0065) (17.3257, -26.9903) (17.3215, -26.9742) (17.3172, -26.9582) (17.313, -26.9422) (17.3087, -26.9263) (17.3044, -26.9104) (17.3002, -26.8947) (17.2959, -26.8789) (17.2916, -26.8633) (17.2872, -26.8477) (17.2829, -26.8322) (17.2786, -26.8167) (17.2742, -26.8013) (17.2699, -26.786) (17.2655, -26.7707) (17.2611, -26.7555) (17.2567, -26.7404) (17.2523, -26.7253) (17.2479, -26.7103) (17.2435, -26.6954) (17.2391, -26.6805) (17.2346, -26.6657) (17.2302, -26.651) (17.2258, -26.6363) (17.2213, -26.6217) (17.2168, -26.6072) (17.2124, -26.5927) (17.2079, -26.5783) (17.2034, -26.564) (17.1989, -26.5498) (17.1944, -26.5356) (17.1899, -26.5215) (17.1854, -26.5074) (17.1809, -26.4935) (17.1764, -26.4796) (17.1719, -26.4658) (17.1674, -26.452) (17.1629, -26.4384) (17.1584, -26.4247) (17.1538, -26.4112) (17.1493, -26.3978) (17.1448, -26.3844) (17.1402, -26.3711) (17.1357, -26.3578) (17.1312, -26.3447) (17.1266, -26.3316) (17.1221, -26.3186) (17.1175, -26.3057) (17.113, -26.2928) (17.1085, -26.2801) (17.1039, -26.2674) (17.0994, -26.2547) (17.0949, -26.2422) (17.0903, -26.2297) (17.0858, -26.2173) (17.0813, -26.205) (17.0768, -26.1928) (17.0723, -26.1807) (17.0677, -26.1686) (17.0632, -26.1566) (17.0587, -26.1447) (17.0542, -26.1329) (17.0497, -26.1212) (17.0452, -26.1095) (17.0408, -26.0979) (17.0363, -26.0864) (17.0318, -26.075) (17.0274, -26.0637) (17.0229, -26.0525) (17.0185, -26.0413) (17.014, -26.0303) (17.0096, -26.0193) (17.0052, -26.0084) (17.0008, -25.9976) (16.9964, -25.9869) (16.992, -25.9763) (16.9877, -25.9657) (16.9833, -25.9553) (16.979, -25.9449) (16.9746, -25.9347) (16.9703, -25.9245) (16.966, -25.9144) (16.9618, -25.9044) (16.9575, -25.8945) (16.9532, -25.8847) (16.949, -25.875) (16.9448, -25.8654) (16.9406, -25.8559) (16.9364, -25.8464) (16.9323, -25.8371) (16.9281, -25.8279) (16.924, -25.8188) (16.9199, -25.8097) (16.9159, -25.8008) (16.9118, -25.792) (16.9078, -25.7832) (16.9038, -25.7746) (16.8998, -25.7661) (16.8959, -25.7576) (16.892, -25.7493) (16.8881, -25.7411) (16.8842, -25.733) (16.8804, -25.725) (16.8766, -25.7171) (16.8728, -25.7093) (16.8691, -25.7016) (16.8654, -25.6941) (16.8617, -25.6866) (16.8581, -25.6792) (16.8545, -25.672) (16.8509, -25.6649) (16.8474, -25.6579) (16.8439, -25.651) (16.8404, -25.6442) (16.837, -25.6376) (16.8337, -25.631) (16.8303, -25.6246) (16.8271, -25.6183) (16.8238, -25.6121) (16.8206, -25.6061) (16.8175, -25.6001) (16.8144, -25.5943) (16.8114, -25.5887) (16.8084, -25.5831) (16.8055, -25.5777) (16.8026, -25.5724) (16.7998, -25.5673) (16.797, -25.5623) (16.7943, -25.5574) (16.7917, -25.5526) (16.7891, -25.548) (16.7866, -25.5436) (16.7841, -25.5392) (16.7817, -25.5351) (16.7794, -25.531) (16.7772, -25.5271) (16.775, -25.5234) (16.7729, -25.5198) (16.7709, -25.5164) (16.769, -25.5131) (16.7672, -25.51) (16.7654, -25.5071) (16.7637, -25.5043) (16.7621, -25.5017) (16.7606, -25.4992) (16.7593, -25.4969) (16.758, -25.4948) (16.7568, -25.4929) (16.7557, -25.4911) (16.7547, -25.4896) (16.7538, -25.4882) (16.7531, -25.487) (16.7526, -25.4862) (16.7523, -25.4857) (16.7521, -25.4854) (16.752, -25.4853) knots -1 -1 -1 -1 -1 -1 -0.99583333 -0.99166667 -0.9875 -0.98333333 -0.97916667 -0.975 -0.97083333 -0.96666667 -0.9625 -0.95833333 -0.95416667 -0.95 -0.94583333 -0.94166667 -0.9375 -0.93333333 -0.92916667 -0.925 -0.92083333 -0.91666667 -0.9125 -0.90833333 -0.90416667 -0.9 -0.89583333 -0.89166667 -0.8875 -0.88333333 -0.87916667 -0.875 -0.87083333 -0.86666667 -0.8625 -0.85833333 -0.85416667 -0.85 -0.84583333 -0.84166667 -0.8375 -0.83333333 -0.82916667 -0.825 -0.82083333 -0.81666667 -0.8125 -0.80833333 -0.80416667 -0.8 -0.79583333 -0.79166667 -0.7875 -0.78333333 -0.77916667 -0.775 -0.77083333 -0.76666667 -0.7625 -0.75833333 -0.75416667 -0.75 -0.74583333 -0.74166667 -0.7375 -0.73333333 -0.72916667 -0.725 -0.72083333 -0.71666667 -0.7125 -0.70833333 -0.70416667 -0.7 -0.69583333 -0.69166667 -0.6875 -0.68333333 -0.67916667 -0.675 -0.67083333 -0.66666667 -0.6625 -0.65833333 -0.65416667 -0.65 -0.64583333 -0.64166667 -0.6375 -0.63333333 -0.62916667 -0.625 -0.62083333 -0.61666667 -0.6125 -0.60833333 -0.60416667 -0.6 -0.59583333 -0.59166667 -0.5875 -0.58333333 -0.57916667 -0.575 -0.57083333 -0.56666667 -0.5625 -0.55833333 -0.55416667 -0.55 -0.54583333 -0.54166667 -0.5375 -0.53333333 -0.52916667 -0.525 -0.52083333 -0.51666667 -0.5125 -0.50833333 -0.50416667 -0.5 -0.49583333 -0.49166667 -0.4875 -0.48333333 -0.47916667 -0.475 -0.47083333 -0.46666667 -0.4625 -0.45833333 -0.45416667 -0.45 -0.44583333 -0.44166667 -0.4375 -0.43333333 -0.42916667 -0.425 -0.42083333 -0.41666667 -0.4125 -0.40833333 -0.40416667 -0.4 -0.39583333 -0.39166667 -0.3875 -0.38333333 -0.37916667 -0.375 -0.37083333 -0.36666667 -0.3625 -0.35833333 -0.35416667 -0.35 -0.34583333 -0.34166667 -0.3375 -0.33333333 -0.32916667 -0.325 -0.32083333 -0.31666667 -0.3125 -0.30833333 -0.30416667 -0.3 -0.29583333 -0.29166667 -0.2875 -0.28333333 -0.27916667 -0.275 -0.27083333 -0.26666667 -0.2625 -0.25833333 -0.25416667 -0.25 -0.24583333 -0.24166667 -0.2375 -0.23333333 -0.22916667 -0.225 -0.22083333 -0.21666667 -0.2125 -0.20833333 -0.20416667 -0.2 -0.19583333 -0.19166667 -0.1875 -0.18333333 -0.17916667 -0.175 -0.17083333 -0.16666667 -0.1625 -0.15833333 -0.15416667 -0.15 -0.14583333 -0.14166667 -0.1375 -0.13333333 -0.12916667 -0.125 -0.12083333 -0.11666667 -0.1125 -0.10833333 -0.10416667 -0.1 -0.09583333 -0.09166667 -0.0875 -0.08333333 -0.07916667 -0.075 -0.07083333 -0.06666667 -0.0625 -0.05833333 -0.05416667 -0.05 -0.04583333 -0.04166667 -0.0375 -0.03333333 -0.02916667 -0.025 -0.02083333 -0.01666667 -0.0125 -0.00833333 -0.00416667 0 0 0 0 0 0
  line L42 (16.752, -25.4853) -> (16.7512, -25.4842)
  line L43 (16.7512, -25.4842) -> (15.8605, -24.129)
  arc A22 (15.8605, -24.129) -> (18.0469, -22.5405) centre (0, 0) ccw
  line L44 (18.0469, -22.5405) -> (19.0605, -23.8064)
  line L45 (19.0605, -23.8064) -> (19.0613, -23.8075)
  spline S22 degree 5 poles (19.0613, -23.8075) (19.0614, -23.8076) (19.0616, -23.8079) (19.062, -23.8083) (19.0626, -23.809) (19.0635, -23.8101) (19.0645, -23.8114) (19.0657, -23.8128) (19.0671, -23.8144) (19.0685, -23.8161) (19.0701, -23.818) (19.0719, -23.82) (19.0737, -23.8222) (19.0757, -23.8245) (19.0779, -23.827) (19.0801, -23.8295) (19.0825, -23.8323) (19.085, -23.8351) (19.0877, -23.8381) (19.0904, -23.8412) (19.0933, -23.8444) (19.0963, -23.8477) (19.0994, -23.8512) (19.1027, -23.8547) (19.106, -23.8584) (19.1095, -23.8621) (19.1131, -23.866) (19.1168, -23.87) (19.1206, -23.8741) (19.1245, -23.8783) (19.1285, -23.8825) (19.1327, -23.8869) (19.1369, -23.8914) (19.1413, -23.8959) (19.1457, -23.9005) (19.1503, -23.9053) (19.155, -23.9101) (19.1597, -23.915) (19.1646, -23.92) (19.1696, -23.925) (19.1747, -23.9302) (19.1798, -23.9354) (19.1851, -23.9407) (19.1905, -23.9461) (19.196, -23.9515) (19.2015, -23.957) (19.2072, -23.9626) (19.213, -23.9683) (19.2188, -23.974) (19.2248, -23.9798) (19.2309, -23.9857) (19.237, -23.9916) (19.2433, -23.9976) (19.2496, -24.0037) (19.256, -24.0098) (19.2625, -24.016) (19.2692, -24.0222) (19.2759, -24.0285) (19.2826, -24.0348) (19.2895, -24.0413) (19.2965, -24.0477) (19.3036, -24.0542) (19.3107, -24.0608) (19.318, -24.0675) (19.3253, -24.0741) (19.3327, -24.0809) (19.3402, -24.0877) (19.3478, -24.0945) (19.3554, -24.1014) (19.3632, -24.1083) (19.371, -24.1153) (19.379, -24.1223) (19.387, -24.1294) (19.3951, -24.1365) (19.4033, -24.1436) (19.4115, -24.1509) (19.4199, -24.1581) (19.4283, -24.1654) (19.4368, -24.1727) (19.4454, -24.1801) (19.4541, -24.1875) (19.4628, -24.1949) (19.4717, -24.2024) (19.4806, -24.2099) (19.4896, -24.2175) (19.4986, -24.2251) (19.5078, -24.2327) (19.517, -24.2404) (19.5263, -24.2481) (19.5357, -24.2559) (19.5452, -24.2636) (19.5547, -24.2714) (19.5643, -24.2793) (19.574, -24.2871) (19.5838, -24.295) (19.5937, -24.303) (19.6036, -24.3109) (19.6136, -24.3189) (19.6237, -24.3269) (19.6338, -24.335) (19.6441, -24.3431) (19.6544, -24.3512) (19.6647, -24.3593) (19.6752, -24.3675) (19.6857, -24.3757) (19.6963, -24.3839) (19.707, -24.3921) (19.7178, -24.4004) (19.7286, -24.4087) (19.7395, -24.417) (19.7504, -24.4253) (19.7615, -24.4337) (19.7726, -24.442) (19.7838, -24.4504) (19.795, -24.4589) (19.8063, -24.4673) (19.8177, -24.4758) (19.8292, -24.4843) (19.8407, -24.4928) (19.8524, -24.5013) (19.864, -24.5098) (19.8758, -24.5184) (19.8876, -24.527) (19.8995, -24.5356) (19.9114, -24.5442) (19.9235, -24.5528) (19.9356, -24.5615) (19.9477, -24.5702) (19.96, -24.5788) (19.9723, -24.5875) (19.9846, -24.5963) (19.9971, -24.605) (20.0096, -24.6137) (20.0221, -24.6225) (20.0348, -24.6313) (20.0475, -24.6401) (20.0603, -24.6489) (20.0731, -24.6577) (20.086, -24.6665) (20.099, -24.6753) (20.112, -24.6842) (20.1251, -24.693) (20.1383, -24.7019) (20.1515, -24.7108) (20.1648, -24.7197) (20.1782, -24.7286) (20.1916, -24.7375) (20.2051, -24.7465) (20.2187, -24.7554) (20.2323, -24.7643) (20.246, -24.7733) (20.2597, -24.7823) (20.2735, -24.7912) (20.2874, -24.8002) (20.3014, -24.8092) (20.3154, -24.8182) (20.3294, -24.8272) (20.3436, -24.8362) (20.3578, -24.8452) (20.372, -24.8542) (20.3864, -24.8633) (20.4007, -24.8723) (20.4152, -24.8813) (20.4297, -24.8904) (20.4443, -24.8994) (20.4589, -24.9085) (20.4736, -24.9176) (20.4883, -24.9266) (20.5032, -24.9357) (20.518, -24.9448) (20.533, -24.9538) (20.548, -24.9629) (20.563, -24.972) (20.5781, -24.9811) (20.5933, -24.9902) (20.6086, -24.9993) (20.6239, -25.0084) (20.6392, -25.0174) (20.6546, -25.0265) (20.6701, -25.0356) (20.6857, -25.0447) (20.7013, -25.0538) (20.7169, -25.0629) (20.7326, -25.072) (20.7484, -25.0811) (20.7642, -25.0902) (20.7801, -25.0993) (20.7961, -25.1084) (20.8121, -25.1175) (20.8281, -25.1266) (20.8443, -25.1357) (20.8605, -25.1448) (20.8767, -25.1539) (20.893, -25.163) (20.9093, -25.1721) (20.9258, -25.1812) (20.9422, -25.1903) (20.9588, -25.1994) (20.9753, -25.2085) (20.992, -25.2175) (21.0087, -25.2266) (21.0254, -25.2357) (21.0422, -25.2448) (21.0591, -25.2538) (21.076, -25.2629) (21.093, -25.2719) (21.11, -25.281) (21.1271, -25.29) (21.1443, -25.2991) (21.1615, -25.3081) (21.1787, -25.3172) (21.196, -25.3262) (21.2134, -25.3352) (21.2308, -25.3442) (21.2483, -25.3533) (21.2658, -25.3623) (21.2834, -25.3713) (21.301, -25.3803) (21.3187, -25.3892) (21.3365, -25.3982) (21.3543, -25.4072) (21.3721, -25.4162) (21.39, -25.4251) (21.408, -25.4341) (21.426, -25.443) (21.4441, -25.452) (21.4622, -25.4609) (21.4804, -25.4698) (21.4986, -25.4787) (21.5169, -25.4876) (21.5352, -25.4965) (21.5536, -25.5054) (21.572, -25.5143) (21.5905, -25.5232) (21.6091, -25.5321) (21.6277, -25.5409) (21.6463, -25.5498) (21.665, -25.5586) (21.6838, -25.5674) (21.7026, -25.5762) (21.7214, -25.585) (21.7365, -25.5921) (21.7479, -25.5973) (21.7555, -25.6009) (21.7593, -25.6026) knots 0 0 0 0 0 0 0.00416667 0.00833333 0.0125 0.01666667 0.02083333 0.025 0.02916667 0.03333333 0.0375 0.04166667 0.04583333 0.05 0.05416667 0.05833333 0.0625 0.06666667 0.07083333 0.075 0.07916667 0.08333333 0.0875 0.09166667 0.09583333 0.1 0.10416667 0.10833333 0.1125 0.11666667 0.12083333 0.125 0.12916667 0.13333333 0.1375 0.14166667 0.14583333 0.15 0.15416667 0.15833333 0.1625 0.16666667 0.17083333 0.175 0.17916667 0.18333333 0.1875 0.19166667 0.19583333 0.2 0.20416667 0.20833333 0.2125 0.21666667 0.22083333 0.225 0.22916667 0.23333333 0.2375 0.24166667 0.24583333 0.25 0.25416667 0.25833333 0.2625 0.26666667 0.27083333 0.275 0.27916667 0.28333333 0.2875 0.29166667 0.29583333 0.3 0.30416667 0.30833333 0.3125 0.31666667 0.32083333 0.325 0.32916667 0.33333333 0.3375 0.34166667 0.34583333 0.35 0.35416667 0.35833333 0.3625 0.36666667 0.37083333 0.375 0.37916667 0.38333333 0.3875 0.39166667 0.39583333 0.4 0.40416667 0.40833333 0.4125 0.41666667 0.42083333 0.425 0.42916667 0.43333333 0.4375 0.44166667 0.44583333 0.45 0.45416667 0.45833333 0.4625 0.46666667 0.47083333 0.475 0.47916667 0.48333333 0.4875 0.49166667 0.49583333 0.5 0.50416667 0.50833333 0.5125 0.51666667 0.52083333 0.525 0.52916667 0.53333333 0.5375 0.54166667 0.54583333 0.55 0.55416667 0.55833333 0.5625 0.56666667 0.57083333 0.575 0.57916667 0.58333333 0.5875 0.59166667 0.59583333 0.6 0.60416667 0.60833333 0.6125 0.61666667 0.62083333 0.625 0.62916667 0.63333333 0.6375 0.64166667 0.64583333 0.65 0.65416667 0.65833333 0.6625 0.66666667 0.67083333 0.675 0.67916667 0.68333333 0.6875 0.69166667 0.69583333 0.7 0.70416667 0.70833333 0.7125 0.71666667 0.72083333 0.725 0.72916667 0.73333333 0.7375 0.74166667 0.74583333 0.75 0.75416667 0.75833333 0.7625 0.76666667 0.77083333 0.775 0.77916667 0.78333333 0.7875 0.79166667 0.79583333 0.8 0.80416667 0.80833333 0.8125 0.81666667 0.82083333 0.825 0.82916667 0.83333333 0.8375 0.84166667 0.84583333 0.85 0.85416667 0.85833333 0.8625 0.86666667 0.87083333 0.875 0.87916667 0.88333333 0.8875 0.89166667 0.89583333 0.9 0.90416667 0.90833333 0.9125 0.91666667 0.92083333 0.925 0.92916667 0.93333333 0.9375 0.94166667 0.94583333 0.95 0.95416667 0.95833333 0.9625 0.96666667 0.97083333 0.975 0.97916667 0.98333333 0.9875 0.99166667 0.99583333 1 1 1 1 1 1
  arc A23 (21.7593, -25.6026) -> (23.1879, -24.3163) centre (0, 0) ccw